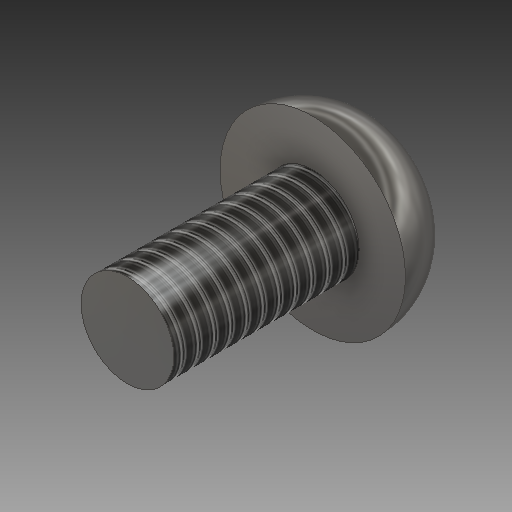
# Autodesk Inventor part: ネジ鍋m4,08
Saved by Autodesk Inventor 2020 (Build 240168000, 168)
## iProperties
Part Number: ネジ鍋m4,08
Material: 鋼、高強度、低合金
Document SubType Name: Modeling
Designer: 雪村
Density: 7.85 g/cm^3
Appearance: 鋼 - つや出し
Mass: 1.67593 g
Surface Area: 2.41259 cm^2
Volume: 0.213495 cm^3
Author: 雪村
Autodesk Inventor part; units mm, degrees
ref_plane "YZ Plane" through (0, 0, 0) normal (1, 0, 0) x (0, 1, 0)
ref_plane "XZ Plane" through (0, 0, 0) normal (0, 1, 0) x (-1, 0, 0)
ref_plane "XY Plane" through (0, 0, 0) normal (0, 0, 1) x (1, 0, 0)
sketch "スケッチ1" plane through (0, 0, 0) normal (0, 0, 1) x (1, 0, 0)
  circle A0 centre (0, 0) radius 2
  dimension "d1" = 4
  constraints: 1 centre point, 1 coincident
  measures "d1" diameter of A0
extrude "押し出し1" add sketch "スケッチ1" along normal blind 8
sketch "スケッチ2" plane through (0, 0, 0) normal (0, 0, -1) x (-1, 0, 0)
  circle A0 centre (0, 0) radius 2 projected
  circle A1 centre (0, 0) radius 4
  dimension "d4" = 8
  constraints: 1 centre point, 1 coincident
  measures "d4" diameter of A1
extrude "押し出し2" add sketch "スケッチ2" along normal blind 3.1 contours A0 | A1
fillet "フィレット1" radius 3.1 1 edges at (4, 0, -3.1)
thread "ねじ1" size "M4x0.7" class "6g" standard "ANSI Metric M Profile" full length
